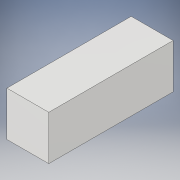
# Autodesk Inventor part: battery
Saved by Autodesk Inventor 2019 (Build 230136000, 136)
## iProperties
Created: 2019-04-07
Part Number: battery
Material: PPS Plastic
Document SubType Name: Modeling
Designer: albaa
Mass: 221.663 g
Surface Area: 176.216 cm^2
Volume: 135.408 cm^3
Density: 1.637 g/cm^3
Appearance: Smooth - White
Author: albaa
Autodesk Inventor part; units mm, degrees
ref_plane "YZ Plane" through (0, 0, 0) normal (1, 0, 0) x (0, 1, 0)
ref_plane "XZ Plane" through (0, 0, 0) normal (0, 1, 0) x (-1, 0, 0)
ref_plane "XY Plane" through (0, 0, 0) normal (0, 0, 1) x (1, 0, 0)
sketch "Sketch1" plane through (0, 0, 0) normal (0, 1, 0) x (-1, 0, 0)
  line L0 (17.5, 52) -> (-17.5, 52)
  line L1 (-17.5, 52) -> (-17.5, -52)
  line L2 (-17.5, -52) -> (17.5, -52)
  line L3 (17.5, -52) -> (17.5, 52)
  line L4 (17.5, 52) -> (-17.5, -52) construction
  line L5 (-17.5, 52) -> (17.5, -52) construction
  point P0 (0, 0)
  dimension "d0" = 104
  dimension "d1" = 35
  constraints: 12 end point, 2 midpoint, 2 parallel, 1 horizontal, 1 perpendicular
  measures "d0" distance of L0.end L1.end
  measures "d1" distance of L1.end L2.end
extrude "Extrusion1" add sketch "Sketch1" along normal blind 18.6 and the other way blind 18.6
body "Solid1"
